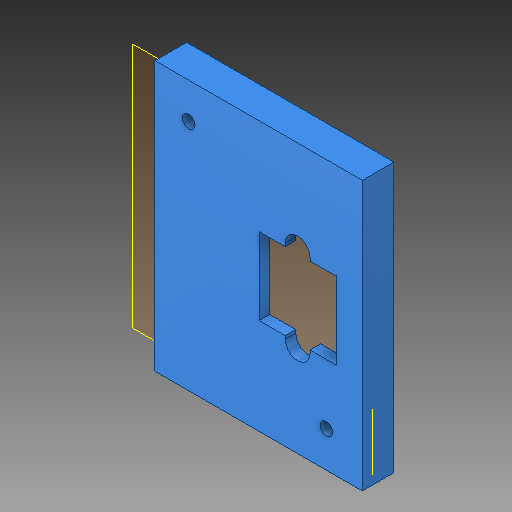
# Autodesk Inventor part: frontCase
Saved by Autodesk Inventor 2017 (Build 210142000, 142)
## iProperties
Created: 2016-12-21
Part Number: frontCase
Material: Generic
Document SubType Name: Modeling
Designer: PLTW
Density: 1 g/cm^3
Appearance: Cyan
Author: PLTW
Autodesk Inventor part; units mm, degrees
ref_plane "YZ Plane" through (0, 0, 0) normal (1, 0, 0) x (0, 1, 0)
ref_plane "XZ Plane" through (0, 0, 0) normal (0, 1, 0) x (-1, 0, 0)
ref_plane "XY Plane" through (0, 0, 0) normal (0, 0, 1) x (1, 0, 0)
ref_plane "Work Plane1" through (0, 0, 0) normal (0, 0, 1) x (1, 0, 0)
sketch "Sketch1" plane through (0, 0, 0) normal (0, 0, 1) x (1, 0, 0)
  line L0 (19.5326, 20.4724) -> (19.5326, 14.097) projected
  line L1 (19.5326, 14.097) -> (13.5636, 14.097) projected
  line L2 (13.5636, 14.097) -> (13.5636, 20.4724) projected
  line L3 (13.5636, 20.4724) -> (19.5326, 20.4724) projected
  line L4 (13.4112, 9.0424) -> (13.4112, 4.2164) projected
  line L5 (13.4112, 4.2164) -> (9.6012, 4.2164) projected
  line L6 (9.6012, 4.2164) -> (9.6012, 9.0424) projected
  line L7 (9.6012, 9.0424) -> (13.4112, 9.0424) projected
  line L8 (13.335, -14.5034) -> (13.335, -17.7038) projected
  line L9 (13.335, -17.7038) -> (8.3566, -17.7038) projected
  line L10 (8.3566, -17.7038) -> (8.3566, -14.5034) projected
  line L11 (8.3566, -14.5034) -> (13.335, -14.5034) projected
  line L12 (24.1808, 3.429) -> (24.1808, -13.589) projected
  line L13 (24.1808, -13.589) -> (7.1628, -13.589) projected
  line L14 (7.1628, -13.589) -> (7.1628, 3.429) projected
  line L15 (7.1628, 3.429) -> (24.1808, 3.429) projected
  line L16 (0.635, -1.7526) -> (0.635, 1.7526) projected
  line L17 (0.635, 1.7526) -> (3.4569, 1.7526) projected
  line L18 (3.4569, 1.7526) -> (3.4569, -1.7526) projected
  line L19 (3.4569, -1.7526) -> (0.635, -1.7526) projected
  arc A0 (35.2933, -10.0203) -> (39.7383, -10.0203) centre (37.5158, -10.0203) ccw projected
  line L20 (35.2933, -10.0203) -> (35.2933, -8.509) projected
  line L21 (35.2933, -8.509) -> (29.0068, -8.509) projected
  line L22 (29.0068, -8.509) -> (29.0068, 8.509) projected
  line L23 (29.0068, 8.509) -> (35.2933, 8.509) projected
  line L24 (35.2933, 8.509) -> (35.2933, 10.0203) projected
  arc A1 (39.7383, 10.0203) -> (35.2933, 10.0203) centre (37.5158, 10.0203) ccw projected
  line L25 (39.7383, 10.0203) -> (39.7383, 8.509) projected
  line L26 (39.7383, 8.509) -> (46.0248, 8.509) projected
  line L27 (46.0248, 8.509) -> (46.0248, -8.509) projected
  line L28 (46.0248, -8.509) -> (39.7383, -8.509) projected
  line L29 (39.7383, -8.509) -> (39.7383, -10.0203) projected
  circle A2 centre (11.303, 23.749) radius 1.524 projected
  circle A3 centre (44.45, -23.749) radius 1.524 projected
  circle A4 centre (44.45, 23.749) radius 1.524 projected
  circle A5 centre (0, -10.414) radius 1.524 projected
  circle A6 centre (0, 10.414) radius 1.524 projected
  line L30 (3.175, 14.224) -> (-3.175, 14.224) projected
  line L31 (-3.175, 14.224) -> (-3.175, -14.224) projected
  line L32 (-3.175, -14.224) -> (3.175, -14.224) projected
  line L33 (3.175, -14.224) -> (3.175, -26.924) projected
  line L34 (3.175, -26.924) -> (47.625, -26.924) projected
  line L35 (47.625, -26.924) -> (47.625, 26.924) projected
  line L36 (47.625, 26.924) -> (3.175, 26.924) projected
  line L37 (3.175, 26.924) -> (3.175, 14.224) projected
  circle A7 centre (44.45, -23.749) radius 1.524
  circle A8 centre (44.45, -23.749) radius 2.794
  circle A9 centre (44.45, 23.749) radius 1.524
  circle A10 centre (11.303, 23.749) radius 1.524
  circle A11 centre (11.303, 23.749) radius 2.794
  point P0 (0, 0)
  dimension "d0" = 1.27
  constraints: 5 centre point, 5 coincident, 4 equal radius
  measures "d0" radial gap between concentric circles of A8 A3
ref_plane "Work Plane2" through (3.175, -9.6012, 2.286) normal (0, 0, 1) x (1, 0, 0)
ref_plane "Work Plane4" through (3.175, -29.845, 3.556) normal (0, 0, 1) x (1, 0, 0)
extrude "Extrusion1" add sketch "Sketch1" along normal up to surface (3.556 mm away) contours A8 | A11
ref_plane "Work Plane3" through (26.8605, -28.575, 1.016) normal (0, 0, 1) x (1, 0, 0)
sketch "Sketch2" plane through (26.8605, -28.575, 1.016) normal (0, 0, 1) x (1, 0, 0)
  line L0 (-7.3279, 49.0474) -> (-7.3279, 42.672) projected
  line L1 (-7.3279, 42.672) -> (-13.2969, 42.672) projected
  line L2 (-13.2969, 42.672) -> (-13.2969, 49.0474) projected
  line L3 (-13.2969, 49.0474) -> (-7.3279, 49.0474) projected
  line L4 (-13.4493, 37.6174) -> (-13.4493, 32.7914) projected
  line L5 (-13.4493, 32.7914) -> (-17.2593, 32.7914) projected
  line L6 (-17.2593, 32.7914) -> (-17.2593, 37.6174) projected
  line L7 (-17.2593, 37.6174) -> (-13.4493, 37.6174) projected
  line L8 (-13.5255, 14.0716) -> (-13.5255, 10.8712) projected
  line L9 (-13.5255, 10.8712) -> (-18.5039, 10.8712) projected
  line L10 (-18.5039, 10.8712) -> (-18.5039, 14.0716) projected
  line L11 (-18.5039, 14.0716) -> (-13.5255, 14.0716) projected
  line L12 (-2.6797, 32.004) -> (-2.6797, 14.986) projected
  line L13 (-2.6797, 14.986) -> (-19.6977, 14.986) projected
  line L14 (-19.6977, 14.986) -> (-19.6977, 32.004) projected
  line L15 (-19.6977, 32.004) -> (-2.6797, 32.004) projected
  line L16 (-26.2255, 26.8224) -> (-26.2255, 30.3276) projected
  line L17 (-26.2255, 30.3276) -> (-23.4036, 30.3276) projected
  line L18 (-23.4036, 30.3276) -> (-23.4036, 26.8224) projected
  line L19 (-23.4036, 26.8224) -> (-26.2255, 26.8224) projected
  arc A0 (8.4328, 18.5547) -> (12.8778, 18.5547) centre (10.6553, 18.5547) ccw projected
  line L20 (8.4328, 18.5547) -> (8.4328, 20.066) projected
  line L21 (8.4328, 20.066) -> (2.1463, 20.066) projected
  line L22 (2.1463, 20.066) -> (2.1463, 37.084) projected
  line L23 (2.1463, 37.084) -> (8.4328, 37.084) projected
  line L24 (8.4328, 37.084) -> (8.4328, 38.5953) projected
  arc A1 (12.8778, 38.5953) -> (8.4328, 38.5953) centre (10.6553, 38.5953) ccw projected
  line L25 (12.8778, 38.5953) -> (12.8778, 37.084) projected
  line L26 (12.8778, 37.084) -> (19.1643, 37.084) projected
  line L27 (19.1643, 37.084) -> (19.1643, 20.066) projected
  line L28 (19.1643, 20.066) -> (12.8778, 20.066) projected
  line L29 (12.8778, 20.066) -> (12.8778, 18.5547) projected
  circle A2 centre (-15.5575, 52.324) radius 1.524 projected
  circle A3 centre (17.5895, 4.826) radius 1.524 projected
  circle A4 centre (17.5895, 52.324) radius 1.524 projected
  circle A5 centre (-26.8605, 18.161) radius 1.524 projected
  circle A6 centre (-26.8605, 38.989) radius 1.524 projected
  line L30 (-23.6855, 42.799) -> (-30.0355, 42.799) projected
  line L31 (-30.0355, 42.799) -> (-30.0355, 14.351) projected
  line L32 (-30.0355, 14.351) -> (-23.6855, 14.351) projected
  line L33 (-23.6855, 14.351) -> (-23.6855, 1.651) projected
  line L34 (-23.6855, 1.651) -> (20.7645, 1.651) projected
  line L35 (20.7645, 1.651) -> (20.7645, 55.499) projected
  line L36 (20.7645, 55.499) -> (-23.6855, 55.499) projected
  line L37 (-23.6855, 55.499) -> (-23.6855, 42.799) projected
  line L38 (23.6855, 58.42) -> (-23.6855, 58.42) projected
  line L39 (-23.6855, 58.42) -> (-23.6855, 55.88) projected
  line L40 (-23.6855, 55.88) -> (21.1455, 55.88) projected
  line L41 (21.1455, 55.88) -> (21.1455, 18.9738) projected
  line L42 (21.1455, 18.9738) -> (23.6855, 18.9738) projected
  line L43 (23.6855, 18.9738) -> (23.6855, 58.42) projected
  line L44 (23.6855, 58.42) -> (-23.6855, 58.42)
  line L45 (-23.6855, 58.42) -> (-23.6855, -1.27)
  line L46 (-23.6855, -1.27) -> (23.6855, -1.27)
  line L47 (23.6855, -1.27) -> (23.6855, 58.42)
  line L48 (21.1455, 1.27) -> (-23.6855, 1.27) projected
  line L49 (-23.6855, 1.27) -> (-23.6855, -1.27) projected
  line L50 (-23.6855, -1.27) -> (23.6855, -1.27) projected
  line L51 (23.6855, -1.27) -> (23.6855, 11.2268) projected
  line L52 (23.6855, 11.2268) -> (21.1455, 11.2268) projected
  line L53 (21.1455, 11.2268) -> (21.1455, 1.27) projected
  line L54 (16.3195, 18.9738) -> (16.3195, 11.2268) projected
  line L55 (16.3195, 11.2268) -> (21.1455, 11.2268) projected
  line L56 (21.1455, 18.9738) -> (16.3195, 18.9738) projected
  line L57 (23.6855, 18.9738) -> (16.3195, 18.9738)
  line L58 (16.3195, 18.9738) -> (16.3195, 11.2268)
  line L59 (16.3195, 11.2268) -> (23.6855, 11.2268)
  line L60 (23.6855, 11.2268) -> (23.6855, 18.9738)
  line L61 (19.1643, 37.084) -> (2.1463, 37.084)
  line L62 (2.1463, 37.084) -> (2.1463, 20.066)
  line L63 (2.1463, 20.066) -> (19.1643, 20.066)
  line L64 (19.1643, 20.066) -> (19.1643, 37.084)
  arc A7 (12.8778, 38.5953) -> (8.4328, 38.5953) centre (10.6553, 38.5953) ccw
  arc A8 (8.4328, 18.5547) -> (12.8778, 18.5547) centre (10.6553, 18.5547) ccw
  line L65 (12.8778, 38.5953) -> (12.8778, 37.084)
  line L66 (8.4328, 38.5953) -> (8.4328, 37.084)
  line L67 (12.8778, 18.5547) -> (12.8778, 20.066)
  line L68 (8.4328, 18.5547) -> (8.4328, 20.066)
  line L69 (26.2255, -3.81) -> (-23.6855, -3.81)
  line L70 (-23.6855, 3.81) -> (14.1919, 3.81)
  line L71 (18.6055, 13.7668) -> (26.2255, 13.7668)
  line L72 (26.2255, 13.7668) -> (26.2255, -3.81)
  line L73 (26.2255, 60.96) -> (-23.6855, 60.96)
  line L74 (-23.6855, 54.5712) -> (13.3939, 54.5712)
  line L75 (20.4146, 16.4338) -> (26.2255, 16.4338)
  line L76 (26.2255, 16.4338) -> (26.2255, 60.96)
  line L77 (-23.6855, 58.42) -> (-23.6855, 60.96)
  line L78 (-23.6855, -1.27) -> (-23.6855, -3.81)
  line L79 (20.4146, 48.1106) -> (22.1496, 48.1106)
  line L80 (22.1496, 48.1106) -> (22.1496, 57.15)
  line L81 (22.1496, 57.15) -> (13.3939, 57.15)
  line L82 (13.3939, 57.15) -> (13.3939, 54.5712)
  line L83 (18.6055, 8.0054) -> (22.1496, 8.0054)
  line L84 (22.1496, 8.0054) -> (22.1496, 0)
  line L85 (22.1496, 0) -> (14.1919, 0)
  line L86 (14.1919, 0) -> (14.1919, 3.81)
  line L87 (18.6055, 8.0054) -> (18.6055, 13.7668)
  line L88 (20.4146, 48.1106) -> (20.4146, 16.4338)
  line L89 (26.2255, 16.4338) -> (23.6855, 16.4338)
  line L90 (23.6855, 16.4338) -> (23.6855, 13.7668)
  line L91 (23.6855, 13.7668) -> (26.2255, 13.7668)
  line L92 (26.2255, 13.7668) -> (26.2255, 16.4338)
  arc A9 (7.6708, 18.5547) -> (13.6398, 18.5547) centre (10.6553, 18.5547) ccw
  line L93 (7.6708, 18.5547) -> (7.6708, 19.304)
  line L94 (7.6708, 19.304) -> (1.3843, 19.304)
  line L95 (1.3843, 19.304) -> (1.3843, 37.846)
  line L96 (1.3843, 37.846) -> (7.6708, 37.846)
  line L97 (7.6708, 37.846) -> (7.6708, 38.5953)
  arc A10 (13.6398, 38.5953) -> (7.6708, 38.5953) centre (10.6553, 38.5953) ccw
  line L98 (13.6398, 38.5953) -> (13.6398, 37.846)
  line L99 (13.6398, 37.846) -> (19.9263, 37.846)
  line L100 (19.9263, 37.846) -> (19.9263, 19.304)
  line L101 (19.9263, 19.304) -> (13.6398, 19.304)
  line L102 (13.6398, 19.304) -> (13.6398, 18.5547)
  point P0 (-26.8605, 28.575)
  dimension "d7" = 2.54
  dimension "d8" = 2.54
  dimension "d11" = 0.762
  constraints: 100 end point, 12 perpendicular, 11 parallel, 8 point on circle, 5 horizontal, 5 point on line, 4 centre point, 2 coincident, 2 tangent, 2 vertical, 13 other
  measures "d7" distance between parallel lines of L47 L76
  measures "d8" distance between parallel lines of L51 L72
  measures "d11" distance between parallel lines of L101 L28
extrude "Extrusion3" add sketch "Sketch2" along normal blind 2.54 contours L0 L1 L2 L3 | L4 L5 L6 L7 | L8 L9 L10 L11 | L12 L13 L14 L15 | L45 L17 L18 L19 | L19 L18 L17 L45 L37 L74 L82 L36 L35 L79 L88 L56 L54 L55 L87 L83 L34 L86 L70 L33 | L70 L86 L34 L33 | L37 L36 L82 L74 | L34 L86 L48 L45 | L45 L40 L82 L36 | L34 L35 L83 L53 L48 L86 | L48 L86 L85 L84 L83 L53 L52 L47 L46 L45 | L82 L40 L41 L79 L35 L36 | L39 L38 L43 L42 L41 L79 L80 L81 L82 L40 | L48 L53 L83 L84 L85 L86 | L46 L47 L71 L72 L69 L78 | L82 L81 L80 L79 L41 L40 | L77 L73 L76 L75 L47 L43 L38 | L83 L87 L55 L35 | L35 L55 L53 L83 | L79 L41 L56 L35 | L35 L56 L88 L79 | L55 L87 L71 L35 | L35 L71 L47 L52 L55 | L56 L42 L47 L75 L35 | L35 L75 L88 L56 | L71 L87 L55 L54 L56 L88 L75 L35 | L35 L75 L47 L71 | L47 L75 L92 L71 | A4
sketch "Sketch3" plane through (26.8605, -28.575, 1.016) normal (0, 0, -1) x (-1, 0, 0)
  line L0 (23.6855, -3.81) -> (-26.2255, -3.81) projected
  line L1 (23.6855, 60.96) -> (23.6855, -3.81) projected
  line L2 (23.6855, -3.81) -> (-26.2255, -3.81) projected
  line L3 (23.6855, -1.2698) -> (-26.2255, -1.2698)
  line L4 (-26.2255, -1.2698) -> (-26.2255, -3.81)
  line L5 (-26.2255, -3.81) -> (23.6855, -3.81)
  line L6 (23.6855, -3.81) -> (23.6855, -1.2698)
  line L7 (-26.2255, -3.81) -> (-26.2255, 60.96) projected
  line L8 (-26.2255, 60.96) -> (23.6855, 60.96) projected
  line L9 (-26.2255, -3.81) -> (-23.6855, -3.81)
  line L10 (-23.6855, -3.81) -> (-23.6855, 60.96)
  line L11 (-23.6855, 60.96) -> (-26.2255, 60.96)
  line L12 (-26.2255, 60.96) -> (-26.2255, -3.81)
  line L13 (-23.6855, 11.2268) -> (-23.6855, -1.27) projected
  line L14 (-14.0843, 5.8166) -> (-14.0843, 11.3538) projected
  line L15 (-14.0843, 11.3538) -> (-4.9403, 11.3538) projected
  line L16 (-4.9403, 11.3538) -> (-4.9403, 5.8166) projected
  line L17 (-4.9403, 5.8166) -> (-14.0843, 5.8166) projected
  line L18 (-16.2553, 51.5874) -> (1.5621, 51.5874) projected
  line L19 (1.5621, 51.5874) -> (1.5621, 41.1734) projected
  line L20 (1.5621, 41.1734) -> (-20.2819, 41.1734) projected
  line L21 (-20.2819, 41.1734) -> (-20.2819, 51.5874) projected
  line L22 (-20.2819, 51.5874) -> (-18.9237, 51.5874) projected
  arc A0 (-16.2553, 51.5874) -> (-18.9237, 51.5874) centre (-17.5895, 52.324) ccw projected
  line L23 (23.6855, 47.1424) -> (23.6855, 58.42) projected
  line L24 (23.6855, 58.42) -> (-23.6855, 58.42) projected
  line L25 (-23.6855, 58.42) -> (-23.6855, 18.9738) projected
  line L26 (-23.6855, 18.9738) -> (-16.3195, 18.9738) projected
  line L27 (-16.3195, 18.9738) -> (-16.3195, 11.2268) projected
  line L28 (-16.3195, 11.2268) -> (-23.6855, 11.2268) projected
  line L29 (-23.6855, 11.2268) -> (-23.6855, -1.27) projected
  line L30 (-23.6855, -1.27) -> (23.6855, -1.27) projected
  line L31 (23.6855, -1.27) -> (23.6855, 40.7162) projected
  line L32 (23.6855, 40.7162) -> (8.2423, 40.7162) projected
  line L33 (8.2423, 40.7162) -> (8.2423, 47.1424) projected
  line L34 (8.2423, 47.1424) -> (23.6855, 47.1424) projected
  line L35 (-26.2255, 60.96) -> (23.6855, 60.96)
  line L36 (23.6855, 60.96) -> (23.6855, 58.42)
  line L37 (23.6855, 58.42) -> (-26.2255, 58.42)
  line L38 (-26.2255, 58.42) -> (-26.2255, 60.96)
  circle A1 centre (-17.5895, 4.826) radius 1.524 projected
  circle A2 centre (15.5575, 52.324) radius 1.524 projected
  point P0 (26.8605, 28.575)
  constraints: 24 end point, 6 parallel, 3 horizontal, 3 perpendicular, 3 point on line
extrude "Extrusion4" add sketch "Sketch3" along normal blind 5.08 contours L0 L10 L3 L1 | L0 L4 L3 L10 | L3 L7 L37 L10 | L7 L8 L10 L37 | L24 L10 L8 L1
equation "\"d8\" = d7"
body "Solid1"
